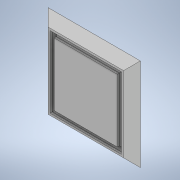
# Autodesk Inventor part: clear-square-notched
Saved by Autodesk Inventor 2021 (Build 250183000, 183)
## iProperties
Created: 2020-12-08
Part Number: clear-square-notched
Material: Generic
Document SubType Name: Modeling
Designer: Luke Kamols
Density: 1 g/cm^3
Appearance: Default
Author: Luke Kamols
Autodesk Inventor part; units mm, degrees
ref_plane "YZ Plane" through (0, 0, 0) normal (1, 0, 0) x (0, 1, 0)
ref_plane "XZ Plane" through (0, 0, 0) normal (0, 1, 0) x (-1, 0, 0)
ref_plane "XY Plane" through (0, 0, 0) normal (0, 0, 1) x (1, 0, 0)
sketch "Sketch1" plane through (0, 0, 0) normal (0, 0, 1) x (1, 0, 0)
  line L0 (0, 0) -> (44, 0)
  line L1 (44, 0) -> (44, 44)
  line L2 (44, 44) -> (0, 44)
  line L3 (0, 44) -> (0, 0)
  dimension "d0" = 44
  dimension "d1" = 44
  constraints: 8 end point, 2 parallel, 1 horizontal, 1 perpendicular
  measures "d0" distance of L2.end L1.end
  measures "d1" distance of L1.end L0.end
extrude "Extrusion1" add sketch "Sketch1" along normal blind 4
chamfer "Chamfer1" distance 4 angle 45 4 edges at (22, 44, 4) (44, 22, 4) (22, 0, 4) (0, 22, 4)
sketch "Sketch2" plane through (0, 0, 4) normal (0, 0, 1) x (1, 0, 0)
  line L0 (40, 4) -> (4, 4) projected
  line L1 (40, 40) -> (40, 4) projected
  line L2 (4, 40) -> (40, 40) projected
  line L3 (4, 4) -> (4, 40) projected
  line L4 (4, 40) -> (40, 40) projected
  line L5 (4, 40) -> (5, 40)
  line L6 (5, 40) -> (5, 39)
  line L7 (5, 39) -> (39, 39)
  line L8 (39, 39) -> (39, 5)
  line L9 (39, 5) -> (5, 5)
  line L10 (5, 5) -> (5, 39)
  line L11 (5, 39) -> (7, 39)
  line L12 (7, 39) -> (7, 37)
  line L13 (7, 37) -> (37, 37)
  line L14 (37, 37) -> (37, 7)
  line L15 (37, 7) -> (7, 7)
  line L16 (7, 7) -> (7, 37)
  point P0 (0, 0)
  dimension "d7" = 1
  dimension "d8" = 1
  dimension "d9" = 34
  dimension "d10" = 34
  dimension "d11" = 2
  dimension "d12" = 2
  dimension "d13" = 30
  dimension "d14" = 30
  constraints: 24 end point, 4 parallel, 4 perpendicular, 2 horizontal, 2 point on line
  measures "d7" distance of L2.start L5.end
  measures "d8" distance of L5.end L6.end
  measures "d9" distance of L8.end L9.end
  measures "d10" distance of L7.end L8.end
  measures "d11" distance of L6.end L11.end
  measures "d12" distance of L11.end L12.end
  measures "d13" distance of L14.end L15.end
  measures "d14" distance of L13.end L14.end
extrude "Extrusion2" cut sketch "Sketch2" against normal blind 2 contours L7 L8 L9 L10
chamfer "Chamfer2" distance 1 angle 45 8 edges at (22, 37, 2) (22, 39, 2) (5, 22, 2) (22, 7, 2) (7, 22, 2) (22, 5, 2) (37, 22, 2) (39, 22, 2)
body "Solid1"
